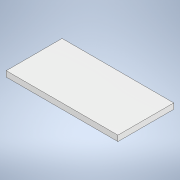
# Autodesk Inventor part: 外置架
Saved by Autodesk Inventor 2020 (Build 240168000, 168)
## iProperties
Created: 2021-04-05
Part Number: 外置架
Material: 聚乙烯，低密度
Document SubType Name: Modeling
Designer: 70929
Density: 0.894 g/cm^3
Appearance: 平滑 - 白色
Author: 70929
Autodesk Inventor part; units mm, degrees
ref_plane "YZ Plane" through (0, 0, 0) normal (1, 0, 0) x (0, 1, 0)
ref_plane "XZ Plane" through (0, 0, 0) normal (0, 1, 0) x (-1, 0, 0)
ref_plane "XY Plane" through (0, 0, 0) normal (0, 0, 1) x (1, 0, 0)
sketch "草图1" plane through (0, 0, 0) normal (0, 1, 0) x (-1, 0, 0)
  line L0 (100, 50) -> (-100, 50)
  line L1 (-100, 50) -> (-100, -50)
  line L2 (-100, -50) -> (100, -50)
  line L3 (100, -50) -> (100, 50)
  line L4 (100, 50) -> (-100, -50) construction
  line L5 (-100, 50) -> (100, -50) construction
  point P0 (0, 0)
  dimension "d0" = 200
  dimension "d1" = 100
  constraints: 12 end point, 2 midpoint, 2 parallel, 1 horizontal, 1 perpendicular
  measures "d0" distance of L2.end L1.end
  measures "d1" distance of L1.end L0.end
extrude "拉伸1" add sketch "草图1" along normal blind 10
